Autodesk Inventor part; units mm, degrees
(part 2 of 2)
  arc A420 (-87.837, 33) -> (-86.5737, 31.4509) centre (-84.0686, 34.7833) ccw
  line L145 (-86.5737, 31.4509) -> (-85.9665, 30.9944)
  arc A421 (-84.6022, 29.6077) -> (-85.9665, 30.9944) centre (-89.9051, 25.7549) ccw
  arc A422 (-85.8476, 25.7748) -> (-84.6022, 29.6077) centre (-86.6173, 28.1437) ccw
  arc A423 (-87.7664, 25.4548) -> (-85.8476, 25.7748) centre (-87.8731, 32.0088) ccw
  line L146 (-87.7664, 25.4548) -> (-88.5259, 25.4425)
  arc A424 (-88.5259, 25.4425) -> (-90.4585, 24.9317) centre (-88.458, 21.274) ccw
  arc A425 (-90.4585, 24.9317) -> (-90.8052, 23.6378) centre (0, 0) ccw
  arc A426 (-90.8052, 23.6378) -> (-89.3869, 22.2292) centre (-87.2439, 25.8052) ccw
  line L147 (-89.3869, 22.2292) -> (-88.7353, 21.8387)
  arc A427 (-87.2336, 20.6022) -> (-88.7353, 21.8387) centre (-92.1048, 16.2162) ccw
  arc A428 (-88.0715, 16.6601) -> (-87.2336, 20.6022) centre (-89.0846, 18.9355) ccw
  arc A429 (-89.9463, 16.1413) -> (-88.0715, 16.6601) centre (-90.7376, 22.6482) ccw
  line L148 (-89.9463, 16.1413) -> (-90.7004, 16.0496)
  arc A430 (-90.7004, 16.0496) -> (-92.5691, 15.3396) centre (-90.1972, 11.9111) ccw
  arc A431 (-92.5691, 15.3396) -> (-92.7786, 14.0166) centre (0, 0) ccw
  arc A432 (-92.7786, 14.0166) -> (-91.2209, 12.7639) centre (-89.4633, 16.5444) ccw
  line L149 (-91.2209, 12.7639) -> (-90.532, 12.4437)
  arc A433 (-88.9092, 11.3709) -> (-90.532, 12.4437) centre (-93.2953, 6.4998) ccw
  arc A434 (-89.3305, 7.3628) -> (-88.9092, 11.3709) centre (-90.5759, 9.5199) ccw
  arc A435 (-91.1408, 6.6509) -> (-89.3305, 7.3628) centre (-92.6079, 13.0394) ccw
  line L150 (-91.1408, 6.6509) -> (-91.8812, 6.4809)
  arc A436 (-91.8812, 6.4809) -> (-93.6654, 5.5795) centre (-90.9481, 2.4177) ccw
  arc A437 (-93.6654, 5.5795) -> (-93.7355, 4.2418) centre (0, 0) ccw
  arc A438 (-93.7355, 4.2418) -> (-92.0553, 3.1588) centre (-90.7026, 7.1023) ccw
  line L151 (-92.0553, 3.1588) -> (-91.3368, 2.9123)
  arc A439 (-89.6108, 2.0151) -> (-91.3368, 2.9123) centre (-93.4636, -3.2878) ccw
  arc A440 (-89.6108, -2.0151) -> (-89.6108, 2.0151) centre (-91.0748, 0) ccw
  arc A441 (-91.3368, -2.9123) -> (-89.6108, -2.0151) centre (-93.4636, 3.2878) ccw
  line L152 (-91.3368, -2.9123) -> (-92.0553, -3.1588)
  arc A442 (-92.0553, -3.1588) -> (-93.7355, -4.2418) centre (-90.7026, -7.1023) ccw
  arc A443 (-93.7355, -4.2418) -> (-93.6654, -5.5795) centre (0, 0) ccw
  arc A444 (-93.6654, -5.5795) -> (-91.8812, -6.4809) centre (-90.9481, -2.4177) ccw
  line L153 (-91.8812, -6.4809) -> (-91.1408, -6.6509)
  arc A445 (-89.3305, -7.3628) -> (-91.1408, -6.6509) centre (-92.6079, -13.0394) ccw
  arc A446 (-88.9092, -11.3709) -> (-89.3305, -7.3628) centre (-90.5759, -9.5199) ccw
  arc A447 (-90.532, -12.4437) -> (-88.9092, -11.3709) centre (-93.2953, -6.4998) ccw
  line L154 (-90.532, -12.4437) -> (-91.2208, -12.7639)
  arc A448 (-91.2208, -12.7639) -> (-92.7786, -14.0166) centre (-89.4633, -16.5443) ccw
  arc A449 (-92.7786, -14.0166) -> (-92.5691, -15.3396) centre (0, 0) ccw
  arc A450 (-92.5691, -15.3396) -> (-90.7004, -16.0496) centre (-90.1972, -11.9111) ccw
  line L155 (-90.7004, -16.0496) -> (-89.9463, -16.1413)
  arc A451 (-88.0715, -16.6601) -> (-89.9463, -16.1413) centre (-90.7376, -22.6482) ccw
  arc A452 (-87.2336, -20.6022) -> (-88.0715, -16.6601) centre (-89.0846, -18.9355) ccw
  arc A453 (-88.7353, -21.8387) -> (-87.2336, -20.6022) centre (-92.1048, -16.2162) ccw
  line L156 (-88.7353, -21.8387) -> (-89.3869, -22.2292)
  arc A454 (-89.3869, -22.2292) -> (-90.8052, -23.6378) centre (-87.2439, -25.8052) ccw
  arc A455 (-90.8052, -23.6378) -> (-90.4585, -24.9317) centre (0, 0) ccw
  arc A456 (-90.4585, -24.9317) -> (-88.5259, -25.4425) centre (-88.458, -21.274) ccw
  line L157 (-88.5259, -25.4425) -> (-87.7664, -25.4548)
  arc A457 (-85.8476, -25.7748) -> (-87.7664, -25.4548) centre (-87.8732, -32.0088) ccw
  arc A458 (-84.6022, -29.6077) -> (-85.8476, -25.7748) centre (-86.6173, -28.1437) ccw
  arc A459 (-85.9665, -30.9944) -> (-84.6022, -29.6077) centre (-89.9052, -25.7549) ccw
  line L158 (-85.9665, -30.9944) -> (-86.5737, -31.4509)
  arc A460 (-86.5737, -31.4509) -> (-87.837, -33) centre (-84.0686, -34.7833) ccw
  arc A461 (-87.837, -33) -> (-87.3569, -34.2506) centre (0, 0) ccw
  arc A462 (-87.3569, -34.2506) -> (-85.3815, -34.5566) centre (-85.7497, -30.4038) ccw
  line L159 (-85.3815, -34.5566) -> (-84.6248, -34.4895)
  arc A463 (-82.6831, -34.6071) -> (-84.6248, -34.4895) centre (-84.0459, -41.0187) ccw
  arc A464 (-81.0439, -38.2889) -> (-82.6831, -34.6071) centre (-83.201, -37.0435) ccw
  arc A465 (-82.2557, -39.8105) -> (-81.0439, -38.2889) centre (-86.7205, -35.0115) ccw
  line L160 (-82.2557, -39.8105) -> (-82.8119, -40.328)
  arc A466 (-82.8119, -40.328) -> (-83.9063, -42.0007) centre (-79.9722, -43.3803) ccw
  arc A467 (-83.9063, -42.0007) -> (-83.2982, -43.1942) centre (0, 0) ccw
  arc A468 (-83.2982, -43.1942) -> (-81.3017, -43.2921) centre (-82.1019, -39.2006) ccw
  line L161 (-81.3017, -43.2921) -> (-80.5561, -43.1462)
  arc A469 (-78.6128, -43.0603) -> (-80.5561, -43.1462) centre (-79.2979, -49.5791) ccw
  arc A470 (-76.5977, -46.5505) -> (-78.6128, -43.0603) centre (-78.8731, -45.5374) ccw
  arc A471 (-77.6438, -48.1905) -> (-76.5977, -46.5505) centre (-82.5858, -43.8844) ccw
  line L162 (-77.6438, -48.1905) -> (-78.1428, -48.7633)
  arc A472 (-78.1428, -48.7633) -> (-79.0564, -50.5412) centre (-74.9996, -51.502) ccw
  arc A473 (-79.0564, -50.5412) -> (-78.3269, -51.6647) centre (0, 0) ccw
  arc A474 (-78.3269, -51.6647) -> (-76.331, -51.5532) centre (-77.5546, -47.5678) ccw
  line L163 (-76.331, -51.5532) -> (-75.6048, -51.3303)
  arc A475 (-73.6811, -51.0416) -> (-75.6048, -51.3303) centre (-73.6811, -57.5964) ccw
  arc A476 (-71.3122, -54.3021) -> (-73.6811, -51.0416) centre (-73.6811, -53.5324) ccw
  arc A477 (-72.1812, -56.0425) -> (-71.3122, -54.3021) centre (-77.5462, -52.2766) ccw
  line L164 (-72.1812, -56.0425) -> (-72.6176, -56.6643)
  arc A478 (-72.6176, -56.6643) -> (-73.3403, -58.528) centre (-69.2054, -59.0595) ccw
  arc A479 (-73.3403, -58.528) -> (-72.4974, -59.569) centre (0, 0) ccw
  arc A480 (-72.4974, -59.569) -> (-70.5241, -59.2496) centre (-72.1575, -55.4139) ccw
  line L165 (-70.5241, -59.2496) -> (-69.8252, -58.9519)
  arc A481 (-67.9421, -58.4638) -> (-69.8252, -58.9519) centre (-67.257, -64.9827) ccw
  arc A482 (-65.2454, -61.4588) -> (-67.9421, -58.4638) centre (-67.6818, -60.9409) ccw
  arc A483 (-65.9277, -63.2805) -> (-65.2454, -61.4588) centre (-71.657, -60.096) ccw
  line L166 (-65.9277, -63.2805) -> (-66.2968, -63.9445)
  arc A484 (-66.2968, -63.9445) -> (-66.8207, -65.8735) centre (-62.6528, -65.9699) ccw
  arc A485 (-66.8207, -65.8735) -> (-65.8735, -66.8207) centre (0, 0) ccw
  arc A486 (-65.8735, -66.8207) -> (-63.9445, -66.2968) centre (-65.9699, -62.6528) ccw
  line L167 (-63.9445, -66.2968) -> (-63.2805, -65.9277)
  arc A487 (-61.4588, -65.2454) -> (-63.2805, -65.9277) centre (-60.096, -71.657) ccw
  arc A488 (-58.4638, -67.9421) -> (-61.4588, -65.2454) centre (-60.941, -67.6818) ccw
  arc A489 (-58.952, -69.8252) -> (-58.4638, -67.9421) centre (-64.9827, -67.257) ccw
  line L168 (-58.952, -69.8252) -> (-59.2496, -70.5241)
  arc A490 (-59.2496, -70.5241) -> (-59.569, -72.4973) centre (-55.4139, -72.1575) ccw
  arc A491 (-59.569, -72.4973) -> (-58.528, -73.3403) centre (0, 0) ccw
  arc A492 (-58.528, -73.3403) -> (-56.6643, -72.6176) centre (-59.0595, -69.2054) ccw
  line L169 (-56.6643, -72.6176) -> (-56.0425, -72.1812)
  arc A493 (-54.3021, -71.3122) -> (-56.0425, -72.1812) centre (-52.2766, -77.5462) ccw
  arc A494 (-51.0416, -73.6811) -> (-54.3021, -71.3122) centre (-53.5324, -73.6811) ccw
  arc A495 (-51.3303, -75.6048) -> (-51.0416, -73.6811) centre (-57.5964, -73.6811) ccw
  line L170 (-51.3303, -75.6048) -> (-51.5532, -76.331)
  arc A496 (-51.5532, -76.331) -> (-51.6647, -78.3269) centre (-47.5678, -77.5545) ccw
  arc A497 (-51.6647, -78.3269) -> (-50.5412, -79.0564) centre (0, 0) ccw
  arc A498 (-50.5412, -79.0564) -> (-48.7633, -78.1428) centre (-51.502, -74.9996) ccw
  line L171 (-48.7633, -78.1428) -> (-48.1905, -77.6438)
  arc A499 (-46.5505, -76.5976) -> (-48.1905, -77.6438) centre (-43.8844, -82.5858) ccw
  arc A500 (-43.0603, -78.6127) -> (-46.5505, -76.5976) centre (-45.5374, -78.8731) ccw
  arc A501 (-43.1462, -80.5561) -> (-43.0603, -78.6127) centre (-49.5792, -79.2979) ccw
  line L172 (-43.1462, -80.5561) -> (-43.2921, -81.3016)
  arc A502 (-43.2921, -81.3016) -> (-43.1943, -83.2982) centre (-39.2006, -82.1019) ccw
  arc A503 (-43.1943, -83.2982) -> (-42.0007, -83.9063) centre (0, 0) ccw
  arc A504 (-42.0007, -83.9063) -> (-40.328, -82.8119) centre (-43.3803, -79.9722) ccw
  line L173 (-40.328, -82.8119) -> (-39.8105, -82.2557)
  arc A505 (-38.2889, -81.0439) -> (-39.8105, -82.2557) centre (-35.0115, -86.7205) ccw
  arc A506 (-34.6071, -82.6831) -> (-38.2889, -81.0439) centre (-37.0435, -83.201) ccw
  arc A507 (-34.4895, -84.6248) -> (-34.6071, -82.6831) centre (-41.0187, -84.0459) ccw
  line L174 (-34.4895, -84.6248) -> (-34.5566, -85.3815)
  arc A508 (-34.5566, -85.3815) -> (-34.2506, -87.3569) centre (-30.4038, -85.7497) ccw
  arc A509 (-34.2506, -87.3569) -> (-33, -87.837) centre (0, 0) ccw
  arc A510 (-33, -87.837) -> (-31.4509, -86.5737) centre (-34.7833, -84.0686) ccw
  line L175 (-31.4509, -86.5737) -> (-30.9944, -85.9665)
  arc A511 (-29.6077, -84.6022) -> (-30.9944, -85.9665) centre (-25.7549, -89.9051) ccw
  arc A512 (-25.7748, -85.8476) -> (-29.6077, -84.6022) centre (-28.1437, -86.6173) ccw
  arc A513 (-25.4548, -87.7664) -> (-25.7748, -85.8476) centre (-32.0088, -87.8731) ccw
  line L176 (-25.4548, -87.7664) -> (-25.4425, -88.5259)
  arc A514 (-25.4425, -88.5259) -> (-24.9317, -90.4585) centre (-21.274, -88.458) ccw
  arc A515 (-24.9317, -90.4585) -> (-23.6378, -90.8052) centre (0, 0) ccw
  arc A516 (-23.6378, -90.8052) -> (-22.2292, -89.3869) centre (-25.8052, -87.2439) ccw
  line L177 (-22.2292, -89.3869) -> (-21.8387, -88.7353)
  arc A517 (-20.6022, -87.2336) -> (-21.8387, -88.7353) centre (-16.2162, -92.1048) ccw
  arc A518 (-16.6601, -88.0715) -> (-20.6022, -87.2336) centre (-18.9355, -89.0846) ccw
  arc A519 (-16.1413, -89.9463) -> (-16.6601, -88.0715) centre (-22.6482, -90.7376) ccw
  line L178 (-16.1413, -89.9463) -> (-16.0496, -90.7004)
  arc A520 (-16.0496, -90.7004) -> (-15.3396, -92.5691) centre (-11.9111, -90.1972) ccw
  arc A521 (-15.3396, -92.5691) -> (-14.0166, -92.7786) centre (0, 0) ccw
  arc A522 (-14.0166, -92.7786) -> (-12.7639, -91.2208) centre (-16.5444, -89.4633) ccw
  line L179 (-12.7639, -91.2208) -> (-12.4437, -90.532)
  arc A523 (-11.3709, -88.9092) -> (-12.4437, -90.532) centre (-6.4998, -93.2952) ccw
  arc A524 (-7.3628, -89.3305) -> (-11.3709, -88.9092) centre (-9.5199, -90.5759) ccw
  arc A525 (-6.6509, -91.1408) -> (-7.3628, -89.3305) centre (-13.0394, -92.6079) ccw
  line L180 (-6.6509, -91.1408) -> (-6.4809, -91.8812)
  arc A526 (-6.4809, -91.8812) -> (-5.5795, -93.6654) centre (-2.4177, -90.9481) ccw
  arc A527 (-5.5795, -93.6654) -> (-4.2418, -93.7355) centre (0, 0) ccw
  arc A528 (-4.2418, -93.7355) -> (-3.1588, -92.0553) centre (-7.1023, -90.7026) ccw
  line L181 (-3.1588, -92.0553) -> (-2.9123, -91.3367)
  arc A529 (-2.0151, -89.6108) -> (-2.9123, -91.3367) centre (3.2878, -93.4636) ccw
  arc A530 (2.0151, -89.6108) -> (-2.0151, -89.6108) centre (0, -91.0748) ccw
  arc A531 (2.9123, -91.3368) -> (2.0151, -89.6108) centre (-3.2879, -93.4636) ccw
  line L182 (2.9123, -91.3368) -> (3.1588, -92.0553)
  arc A532 (3.1588, -92.0553) -> (4.2418, -93.7355) centre (7.1022, -90.7026) ccw
  arc A533 (4.2418, -93.7355) -> (5.5795, -93.6654) centre (0, 0) ccw
  arc A534 (5.5795, -93.6654) -> (6.4809, -91.8812) centre (2.4177, -90.9481) ccw
  line L183 (6.4809, -91.8812) -> (6.6509, -91.1408)
  arc A535 (7.3628, -89.3305) -> (6.6509, -91.1408) centre (13.0394, -92.6079) ccw
  arc A536 (11.3709, -88.9092) -> (7.3628, -89.3305) centre (9.5199, -90.5759) ccw
  arc A537 (12.4436, -90.532) -> (11.3709, -88.9092) centre (6.4998, -93.2952) ccw
  line L184 (12.4436, -90.532) -> (12.7639, -91.2208)
  arc A538 (12.7639, -91.2208) -> (14.0166, -92.7786) centre (16.5443, -89.4633) ccw
  arc A539 (14.0166, -92.7786) -> (15.3396, -92.5691) centre (0, 0) ccw
  arc A540 (15.3396, -92.5691) -> (16.0496, -90.7004) centre (11.9111, -90.1972) ccw
  line L185 (16.0496, -90.7004) -> (16.1413, -89.9463)
  arc A541 (16.6601, -88.0715) -> (16.1413, -89.9463) centre (22.6482, -90.7376) ccw
  arc A542 (20.6022, -87.2336) -> (16.6601, -88.0715) centre (18.9355, -89.0846) ccw
  arc A543 (21.8387, -88.7353) -> (20.6022, -87.2336) centre (16.2162, -92.1048) ccw
  line L186 (21.8387, -88.7353) -> (22.2291, -89.3869)
  arc A544 (22.2291, -89.3869) -> (23.6378, -90.8052) centre (25.8052, -87.2439) ccw
  arc A545 (23.6378, -90.8052) -> (24.9317, -90.4585) centre (0, 0) ccw
  arc A546 (24.9317, -90.4585) -> (25.4424, -88.5259) centre (21.274, -88.458) ccw
  line L187 (25.4424, -88.5259) -> (25.4548, -87.7664)
  arc A547 (25.7748, -85.8476) -> (25.4548, -87.7664) centre (32.0088, -87.8731) ccw
  arc A548 (29.6077, -84.6022) -> (25.7748, -85.8476) centre (28.1437, -86.6173) ccw
  arc A549 (30.9944, -85.9665) -> (29.6077, -84.6022) centre (25.7549, -89.9051) ccw
  line L188 (30.9944, -85.9665) -> (31.4508, -86.5737)
  arc A550 (31.4508, -86.5737) -> (33, -87.837) centre (34.7833, -84.0686) ccw
  arc A551 (33, -87.837) -> (34.2506, -87.3569) centre (0, 0) ccw
  arc A552 (34.2506, -87.3569) -> (34.5566, -85.3815) centre (30.4038, -85.7497) ccw
  line L189 (34.5566, -85.3815) -> (34.4895, -84.6248)
  arc A553 (34.6071, -82.6831) -> (34.4895, -84.6248) centre (41.0187, -84.0459) ccw
  arc A554 (38.2889, -81.0439) -> (34.6071, -82.6831) centre (37.0435, -83.201) ccw
  arc A555 (39.8105, -82.2557) -> (38.2889, -81.0439) centre (35.0115, -86.7205) ccw
  line L190 (39.8105, -82.2557) -> (40.328, -82.8119)
  arc A556 (40.328, -82.8119) -> (42.0007, -83.9063) centre (43.3803, -79.9722) ccw
  arc A557 (42.0007, -83.9063) -> (43.1942, -83.2982) centre (0, 0) ccw
  arc A558 (43.1942, -83.2982) -> (43.292, -81.3017) centre (39.2006, -82.1019) ccw
  line L191 (43.292, -81.3017) -> (43.1462, -80.5561)
  arc A559 (43.0602, -78.6127) -> (43.1462, -80.5561) centre (49.5791, -79.2979) ccw
  arc A560 (46.5505, -76.5976) -> (43.0602, -78.6127) centre (45.5374, -78.8731) ccw
  arc A561 (48.1905, -77.6438) -> (46.5505, -76.5976) centre (43.8844, -82.5858) ccw
  line L192 (48.1905, -77.6438) -> (48.7633, -78.1428)
  arc A562 (48.7633, -78.1428) -> (50.5412, -79.0564) centre (51.502, -74.9996) ccw
  arc A563 (50.5412, -79.0564) -> (51.6646, -78.3269) centre (0, 0) ccw
  arc A564 (51.6646, -78.3269) -> (51.5532, -76.331) centre (47.5678, -77.5546) ccw
  line L193 (51.5532, -76.331) -> (51.3303, -75.6048)
  arc A565 (51.0416, -73.6811) -> (51.3303, -75.6048) centre (57.5964, -73.6811) ccw
  arc A566 (54.3021, -71.3122) -> (51.0416, -73.6811) centre (53.5324, -73.6811) ccw
  arc A567 (56.0425, -72.1812) -> (54.3021, -71.3122) centre (52.2766, -77.5462) ccw
  line L194 (56.0425, -72.1812) -> (56.6643, -72.6176)
  arc A568 (56.6643, -72.6176) -> (58.528, -73.3403) centre (59.0595, -69.2054) ccw
  arc A569 (58.528, -73.3403) -> (59.569, -72.4973) centre (0, 0) ccw
  arc A570 (59.569, -72.4973) -> (59.2496, -70.5241) centre (55.4139, -72.1575) ccw
  line L195 (59.2496, -70.5241) -> (58.9519, -69.8252)
  arc A571 (58.4638, -67.9421) -> (58.9519, -69.8252) centre (64.9827, -67.257) ccw
  arc A572 (61.4588, -65.2454) -> (58.4638, -67.9421) centre (60.9409, -67.6818) ccw
  arc A573 (63.2805, -65.9277) -> (61.4588, -65.2454) centre (60.096, -71.657) ccw
  line L196 (63.2805, -65.9277) -> (63.9445, -66.2968)
  arc A574 (63.9445, -66.2968) -> (65.8735, -66.8207) centre (65.9699, -62.6528) ccw
  arc A575 (65.8735, -66.8207) -> (66.8207, -65.8735) centre (0, 0) ccw
  arc A576 (66.8207, -65.8735) -> (66.2968, -63.9445) centre (62.6528, -65.9699) ccw
  line L197 (66.2968, -63.9445) -> (65.9277, -63.2805)
  arc A577 (65.2454, -61.4588) -> (65.9277, -63.2805) centre (71.657, -60.096) ccw
  arc A578 (67.9421, -58.4638) -> (65.2454, -61.4588) centre (67.6818, -60.941) ccw
  arc A579 (69.8252, -58.9519) -> (67.9421, -58.4638) centre (67.257, -64.9827) ccw
  line L198 (69.8252, -58.9519) -> (70.5241, -59.2496)
  arc A580 (70.5241, -59.2496) -> (72.4973, -59.569) centre (72.1575, -55.4139) ccw
  arc A581 (72.4973, -59.569) -> (73.3403, -58.528) centre (0, 0) ccw
  arc A582 (73.3403, -58.528) -> (72.6176, -56.6643) centre (69.2053, -59.0595) ccw
  line L199 (72.6176, -56.6643) -> (72.1812, -56.0425)
  arc A583 (71.3122, -54.3021) -> (72.1812, -56.0425) centre (77.5462, -52.2766) ccw
  arc A584 (73.6811, -51.0416) -> (71.3122, -54.3021) centre (73.6811, -53.5324) ccw
  arc A585 (75.6048, -51.3303) -> (73.6811, -51.0416) centre (73.6811, -57.5964) ccw
  line L200 (75.6048, -51.3303) -> (76.331, -51.5532)
  arc A586 (76.331, -51.5532) -> (78.3268, -51.6647) centre (77.5545, -47.5678) ccw
  arc A587 (78.3268, -51.6647) -> (79.0564, -50.5412) centre (0, 0) ccw
  arc A588 (79.0564, -50.5412) -> (78.1428, -48.7633) centre (74.9996, -51.502) ccw
  line L201 (78.1428, -48.7633) -> (77.6438, -48.1905)
  arc A589 (76.5976, -46.5505) -> (77.6438, -48.1905) centre (82.5857, -43.8844) ccw
  arc A590 (78.6127, -43.0603) -> (76.5976, -46.5505) centre (78.8731, -45.5374) ccw
  arc A591 (80.5561, -43.1462) -> (78.6127, -43.0603) centre (79.2979, -49.5791) ccw
  line L202 (80.5561, -43.1462) -> (81.3016, -43.2921)
  arc A592 (81.3016, -43.2921) -> (83.2982, -43.1943) centre (82.1019, -39.2006) ccw
  arc A593 (83.2982, -43.1943) -> (83.9063, -42.0007) centre (0, 0) ccw
  arc A594 (83.9063, -42.0007) -> (82.8119, -40.328) centre (79.9722, -43.3803) ccw
  line L203 (82.8119, -40.328) -> (82.2557, -39.8105)
  arc A595 (81.0439, -38.2889) -> (82.2557, -39.8105) centre (86.7205, -35.0115) ccw
  arc A596 (82.6831, -34.6071) -> (81.0439, -38.2889) centre (83.201, -37.0435) ccw
  arc A597 (84.6248, -34.4895) -> (82.6831, -34.6071) centre (84.0459, -41.0187) ccw
  line L204 (84.6248, -34.4895) -> (85.3815, -34.5566)
  arc A598 (85.3815, -34.5566) -> (87.3569, -34.2506) centre (85.7497, -30.4038) ccw
  arc A599 (87.3569, -34.2506) -> (87.837, -33) centre (0, 0) ccw
  arc A600 (87.837, -33) -> (86.5737, -31.4509) centre (84.0686, -34.7833) ccw
  line L205 (86.5737, -31.4509) -> (85.9664, -30.9944)
  arc A601 (84.6022, -29.6077) -> (85.9664, -30.9944) centre (89.9051, -25.7549) ccw
  arc A602 (85.8476, -25.7748) -> (84.6022, -29.6077) centre (86.6173, -28.1437) ccw
  arc A603 (87.7664, -25.4548) -> (85.8476, -25.7748) centre (87.8731, -32.0088) ccw
  line L206 (87.7664, -25.4548) -> (88.5259, -25.4425)
  arc A604 (88.5259, -25.4425) -> (90.4585, -24.9317) centre (88.458, -21.274) ccw
  arc A605 (90.4585, -24.9317) -> (90.8052, -23.6378) centre (0, 0) ccw
  arc A606 (90.8052, -23.6378) -> (89.3869, -22.2292) centre (87.2439, -25.8052) ccw
  line L207 (89.3869, -22.2292) -> (88.7353, -21.8387)
  arc A607 (87.2336, -20.6022) -> (88.7353, -21.8387) centre (92.1048, -16.2162) ccw
  arc A608 (88.0715, -16.6601) -> (87.2336, -20.6022) centre (89.0846, -18.9355) ccw
  arc A609 (89.9463, -16.1413) -> (88.0715, -16.6601) centre (90.7376, -22.6482) ccw
  line L208 (89.9463, -16.1413) -> (90.7004, -16.0496)
  arc A610 (90.7004, -16.0496) -> (92.569, -15.3396) centre (90.1972, -11.9111) ccw
  arc A611 (92.569, -15.3396) -> (92.7786, -14.0166) centre (0, 0) ccw
  arc A612 (92.7786, -14.0166) -> (91.2208, -12.7639) centre (89.4633, -16.5444) ccw
  line L209 (91.2208, -12.7639) -> (90.532, -12.4437)
  arc A613 (88.9092, -11.3709) -> (90.532, -12.4437) centre (93.2952, -6.4998) ccw
  arc A614 (89.3305, -7.3628) -> (88.9092, -11.3709) centre (90.5759, -9.5199) ccw
  arc A615 (91.1408, -6.6509) -> (89.3305, -7.3628) centre (92.6079, -13.0394) ccw
  line L210 (91.1408, -6.6509) -> (91.8812, -6.4809)
  arc A616 (91.8812, -6.4809) -> (93.6654, -5.5795) centre (90.9481, -2.4177) ccw
  arc A617 (93.6654, -5.5795) -> (93.7355, -4.2418) centre (0, 0) ccw
  arc A618 (93.7355, -4.2418) -> (92.0553, -3.1588) centre (90.7026, -7.1023) ccw
  line L211 (92.0553, -3.1588) -> (91.3367, -2.9123)
  arc A619 (89.6108, -2.0151) -> (91.3367, -2.9123) centre (93.4636, 3.2878) ccw
  arc A620 (89.6108, 2.0151) -> (89.6108, -2.0151) centre (91.0748, 0) ccw
  arc A621 (91.3368, 2.9123) -> (89.6108, 2.0151) centre (93.4636, -3.2878) ccw
  line L212 (91.3368, 2.9123) -> (92.0553, 3.1588)
  arc A622 (92.0553, 3.1588) -> (93.7355, 4.2418) centre (90.7026, 7.1022) ccw
  arc A623 (93.7355, 4.2418) -> (93.6654, 5.5795) centre (0, 0) ccw
  arc A624 (93.6654, 5.5795) -> (91.8812, 6.4809) centre (90.9481, 2.4177) ccw
  line L213 (91.8812, 6.4809) -> (91.1408, 6.6509)
  arc A625 (89.3305, 7.3628) -> (91.1408, 6.6509) centre (92.6079, 13.0394) ccw
  arc A626 (88.9092, 11.3709) -> (89.3305, 7.3628) centre (90.5759, 9.5199) ccw
  arc A627 (90.532, 12.4437) -> (88.9092, 11.3709) centre (93.2952, 6.4998) ccw
  line L214 (90.532, 12.4437) -> (91.2208, 12.7639)
  arc A628 (91.2208, 12.7639) -> (92.7786, 14.0166) centre (89.4633, 16.5443) ccw
  arc A629 (92.7786, 14.0166) -> (92.569, 15.3396) centre (0, 0) ccw
  arc A630 (92.569, 15.3396) -> (90.7004, 16.0496) centre (90.1972, 11.9111) ccw
  line L215 (90.7004, 16.0496) -> (89.9463, 16.1413)
  arc A631 (88.0715, 16.6601) -> (89.9463, 16.1413) centre (90.7376, 22.6482) ccw
  arc A632 (87.2336, 20.6022) -> (88.0715, 16.6601) centre (89.0846, 18.9355) ccw
  arc A633 (88.7353, 21.8387) -> (87.2336, 20.6022) centre (92.1048, 16.2162) ccw
  line L216 (88.7353, 21.8387) -> (89.3869, 22.2291)
  arc A634 (89.3869, 22.2291) -> (90.8052, 23.6378) centre (87.2439, 25.8052) ccw
  arc A635 (90.8052, 23.6378) -> (90.4585, 24.9317) centre (0, 0) ccw
  arc A636 (90.4585, 24.9317) -> (88.5259, 25.4425) centre (88.458, 21.274) ccw
  line L217 (88.5259, 25.4425) -> (87.7664, 25.4548)
  arc A637 (85.8476, 25.7748) -> (87.7664, 25.4548) centre (87.8731, 32.0088) ccw
  arc A638 (84.6022, 29.6077) -> (85.8476, 25.7748) centre (86.6173, 28.1437) ccw
  arc A639 (85.9665, 30.9944) -> (84.6022, 29.6077) centre (89.9051, 25.7549) ccw
  line L218 (85.9665, 30.9944) -> (86.5737, 31.4509)
  arc A640 (86.5737, 31.4509) -> (87.837, 33) centre (84.0686, 34.7833) ccw
  arc A641 (87.837, 33) -> (87.3569, 34.2506) centre (0, 0) ccw
  arc A642 (87.3569, 34.2506) -> (85.3815, 34.5566) centre (85.7497, 30.4038) ccw
  line L219 (85.3815, 34.5566) -> (84.6248, 34.4895)
  arc A643 (82.6831, 34.6071) -> (84.6248, 34.4895) centre (84.0459, 41.0187) ccw
  arc A644 (81.0439, 38.2889) -> (82.6831, 34.6071) centre (83.201, 37.0435) ccw
  arc A645 (82.2557, 39.8105) -> (81.0439, 38.2889) centre (86.7205, 35.0115) ccw
  line L220 (82.2557, 39.8105) -> (82.8119, 40.328)
  arc A646 (82.8119, 40.328) -> (83.9063, 42.0007) centre (79.9722, 43.3803) ccw
  arc A647 (83.9063, 42.0007) -> (83.2982, 43.1942) centre (0, 0) ccw
  arc A648 (83.2982, 43.1942) -> (81.3016, 43.2921) centre (82.1019, 39.2006) ccw
  line L221 (81.3016, 43.2921) -> (80.5561, 43.1462)
  arc A649 (78.6127, 43.0603) -> (80.5561, 43.1462) centre (79.2979, 49.5791) ccw
  arc A650 (76.5976, 46.5505) -> (78.6127, 43.0603) centre (78.8731, 45.5374) ccw
  arc A651 (77.6438, 48.1905) -> (76.5976, 46.5505) centre (82.5858, 43.8844) ccw
  line L222 (77.6438, 48.1905) -> (78.1428, 48.7633)
  arc A652 (78.1428, 48.7633) -> (79.0564, 50.5412) centre (74.9996, 51.502) ccw
  arc A653 (79.0564, 50.5412) -> (78.3269, 51.6647) centre (0, 0) ccw
  arc A654 (78.3269, 51.6647) -> (76.331, 51.5532) centre (77.5545, 47.5678) ccw
  line L223 (76.331, 51.5532) -> (75.6048, 51.3303)
  arc A655 (73.6811, 51.0416) -> (75.6048, 51.3303) centre (73.6811, 57.5964) ccw
  arc A656 (71.3122, 54.3021) -> (73.6811, 51.0416) centre (73.6811, 53.5324) ccw
  arc A657 (72.1812, 56.0425) -> (71.3122, 54.3021) centre (77.5462, 52.2766) ccw
  line L224 (72.1812, 56.0425) -> (72.6176, 56.6643)
  arc A658 (72.6176, 56.6643) -> (73.3403, 58.528) centre (69.2053, 59.0595) ccw
  arc A659 (73.3403, 58.528) -> (72.4973, 59.569) centre (0, 0) ccw
  arc A660 (72.4973, 59.569) -> (70.5241, 59.2496) centre (72.1575, 55.4139) ccw
  line L225 (70.5241, 59.2496) -> (69.8251, 58.9519)
  arc A661 (67.9421, 58.4638) -> (69.8251, 58.9519) centre (67.257, 64.9827) ccw
  arc A662 (65.2454, 61.4588) -> (67.9421, 58.4638) centre (67.6818, 60.9409) ccw
  arc A663 (65.9277, 63.2805) -> (65.2454, 61.4588) centre (71.657, 60.096) ccw
  line L226 (65.9277, 63.2805) -> (66.2968, 63.9445)
  arc A664 (66.2968, 63.9445) -> (66.8207, 65.8735) centre (62.6528, 65.9699) ccw
  arc A665 (66.8207, 65.8735) -> (65.8735, 66.8207) centre (0, 0) ccw
  arc A666 (65.8735, 66.8207) -> (63.9445, 66.2968) centre (65.9699, 62.6528) ccw
  line L227 (63.9445, 66.2968) -> (63.2805, 65.9277)
  arc A667 (61.4588, 65.2454) -> (63.2805, 65.9277) centre (60.096, 71.657) ccw
  arc A668 (58.4638, 67.9421) -> (61.4588, 65.2454) centre (60.9409, 67.6818) ccw
  arc A669 (58.9519, 69.8252) -> (58.4638, 67.9421) centre (64.9827, 67.257) ccw
  line L228 (58.9519, 69.8252) -> (59.2496, 70.5241)
  arc A670 (59.2496, 70.5241) -> (59.569, 72.4973) centre (55.4139, 72.1575) ccw
  arc A671 (59.569, 72.4973) -> (58.528, 73.3403) centre (0, 0) ccw
  arc A672 (58.528, 73.3403) -> (56.6643, 72.6176) centre (59.0595, 69.2053) ccw
  line L229 (56.6643, 72.6176) -> (56.0425, 72.1812)
  arc A673 (54.3021, 71.3122) -> (56.0425, 72.1812) centre (52.2766, 77.5462) ccw
  arc A674 (51.0416, 73.6811) -> (54.3021, 71.3122) centre (53.5324, 73.6811) ccw
  arc A675 (51.3303, 75.6048) -> (51.0416, 73.6811) centre (57.5964, 73.6811) ccw
  line L230 (51.3303, 75.6048) -> (51.5532, 76.331)
  arc A676 (51.5532, 76.331) -> (51.6647, 78.3269) centre (47.5678, 77.5545) ccw
  arc A677 (51.6647, 78.3269) -> (50.5412, 79.0564) centre (0, 0) ccw
  arc A678 (50.5412, 79.0564) -> (48.7633, 78.1428) centre (51.502, 74.9996) ccw
  line L231 (48.7633, 78.1428) -> (48.1905, 77.6438)
  arc A679 (46.5505, 76.5976) -> (48.1905, 77.6438) centre (43.8844, 82.5858) ccw
  arc A680 (43.0603, 78.6127) -> (46.5505, 76.5976) centre (45.5374, 78.8731) ccw
  arc A681 (43.1462, 80.5561) -> (43.0603, 78.6127) centre (49.5791, 79.2979) ccw
  line L232 (43.1462, 80.5561) -> (43.292, 81.3016)
  arc A682 (43.292, 81.3016) -> (43.1942, 83.2982) centre (39.2006, 82.1019) ccw
  arc A683 (43.1942, 83.2982) -> (42.0007, 83.9063) centre (0, 0) ccw
  arc A684 (42.0007, 83.9063) -> (40.328, 82.8119) centre (43.3803, 79.9722) ccw
  line L233 (40.328, 82.8119) -> (39.8105, 82.2557)
  arc A685 (38.2889, 81.0439) -> (39.8105, 82.2557) centre (35.0115, 86.7205) ccw
  arc A686 (34.6071, 82.6831) -> (38.2889, 81.0439) centre (37.0435, 83.201) ccw
  arc A687 (34.4895, 84.6248) -> (34.6071, 82.6831) centre (41.0187, 84.0459) ccw
  line L234 (34.4895, 84.6248) -> (34.5566, 85.3815)
  arc A688 (34.5566, 85.3815) -> (34.2506, 87.3569) centre (30.4038, 85.7497) ccw
  arc A689 (34.2506, 87.3569) -> (33, 87.837) centre (0, 0) ccw
  arc A690 (33, 87.837) -> (31.4509, 86.5737) centre (34.7833, 84.0686) ccw
  line L235 (31.4509, 86.5737) -> (30.9944, 85.9665)
  arc A691 (29.6077, 84.6022) -> (30.9944, 85.9665) centre (25.7549, 89.9051) ccw
  arc A692 (25.7748, 85.8476) -> (29.6077, 84.6022) centre (28.1437, 86.6173) ccw
  arc A693 (25.4548, 87.7664) -> (25.7748, 85.8476) centre (32.0088, 87.8731) ccw
  line L236 (25.4548, 87.7664) -> (25.4425, 88.5259)
  arc A694 (25.4425, 88.5259) -> (24.9317, 90.4585) centre (21.274, 88.458) ccw
  arc A695 (24.9317, 90.4585) -> (23.6378, 90.8052) centre (0, 0) ccw
  arc A696 (23.6378, 90.8052) -> (22.2292, 89.3869) centre (25.8052, 87.2439) ccw
  line L237 (22.2292, 89.3869) -> (21.8386, 88.7353)
  arc A697 (20.6022, 87.2336) -> (21.8386, 88.7353) centre (16.2162, 92.1048) ccw
  arc A698 (16.6601, 88.0715) -> (20.6022, 87.2336) centre (18.9355, 89.0846) ccw
  arc A699 (16.1413, 89.9463) -> (16.6601, 88.0715) centre (22.6482, 90.7376) ccw
  line L238 (16.1413, 89.9463) -> (16.0496, 90.7004)
  arc A700 (16.0496, 90.7004) -> (15.3396, 92.5691) centre (11.9111, 90.1972) ccw
  arc A701 (15.3396, 92.5691) -> (14.0166, 92.7786) centre (0, 0) ccw
  arc A702 (14.0166, 92.7786) -> (12.7639, 91.2208) centre (16.5443, 89.4633) ccw
  line L239 (12.7639, 91.2208) -> (12.4436, 90.532)
  arc A703 (11.3709, 88.9092) -> (12.4436, 90.532) centre (6.4998, 93.2952) ccw
  arc A704 (7.3628, 89.3305) -> (11.3709, 88.9092) centre (9.5199, 90.5759) ccw
  arc A705 (6.6509, 91.1408) -> (7.3628, 89.3305) centre (13.0394, 92.6079) ccw
  line L240 (6.6509, 91.1408) -> (6.4809, 91.8812)
  arc A706 (6.4809, 91.8812) -> (5.5795, 93.6654) centre (2.4177, 90.9481) ccw
  arc A707 (5.5795, 93.6654) -> (4.2418, 93.7355) centre (0, 0) ccw
  arc A708 (4.2418, 93.7355) -> (3.1588, 92.0553) centre (7.1022, 90.7026) ccw
  line L241 (3.1588, 92.0553) -> (2.9123, 91.3367)
  arc A709 (2.0151, 89.6108) -> (2.9123, 91.3367) centre (-3.2878, 93.4636) ccw
  arc A710 (-2.0151, 89.6108) -> (2.0151, 89.6108) centre (0, 91.0748) ccw
  arc A711 (-2.9123, 91.3368) -> (-2.0151, 89.6108) centre (3.2878, 93.4636) ccw
  line L242 (-2.9123, 91.3368) -> (-3.1588, 92.0553)
  arc A712 (-3.1588, 92.0553) -> (-4.2418, 93.7355) centre (-7.1023, 90.7026) ccw
  arc A713 (-4.2418, 93.7355) -> (-5.5795, 93.6654) centre (0, 0) ccw
  arc A714 (-5.5795, 93.6654) -> (-6.4809, 91.8812) centre (-2.4177, 90.9481) ccw
  line L243 (-6.4809, 91.8812) -> (-6.6509, 91.1408)
  arc A715 (-7.3628, 89.3305) -> (-6.6509, 91.1408) centre (-13.0394, 92.6079) ccw
  arc A716 (-11.3709, 88.9092) -> (-7.3628, 89.3305) centre (-9.5199, 90.5759) ccw
  arc A717 (-12.4437, 90.532) -> (-11.3709, 88.9092) centre (-6.4998, 93.2952) ccw
  line L244 (-12.4437, 90.532) -> (-12.7639, 91.2208)
  arc A718 (-12.7639, 91.2208) -> (-14.0166, 92.7786) centre (-16.5444, 89.4633) ccw
  arc A719 (-14.0166, 92.7786) -> (-15.3396, 92.5691) centre (0, 0) ccw
  arc A720 (-15.3396, 92.5691) -> (-16.0496, 90.7004) centre (-11.9111, 90.1972) ccw
  line L245 (-16.0496, 90.7004) -> (-16.1413, 89.9463)
  arc A721 (-16.6601, 88.0715) -> (-16.1413, 89.9463) centre (-22.6482, 90.7376) ccw
  arc A722 (-20.6022, 87.2336) -> (-16.6601, 88.0715) centre (-18.9355, 89.0846) ccw
  arc A723 (-21.8387, 88.7353) -> (-20.6022, 87.2336) centre (-16.2162, 92.1048) ccw
  line L246 (-21.8387, 88.7353) -> (-22.2292, 89.3869)
  arc A724 (-22.2292, 89.3869) -> (-23.6378, 90.8052) centre (-25.8052, 87.2439) ccw
  arc A725 (-23.6378, 90.8052) -> (-24.9317, 90.4585) centre (0, 0) ccw
  arc A726 (-24.9317, 90.4585) -> (-25.4425, 88.5259) centre (-21.274, 88.458) ccw
  line L247 (-25.4425, 88.5259) -> (-25.4548, 87.7664)
  arc A727 (-25.7748, 85.8476) -> (-25.4548, 87.7664) centre (-32.0088, 87.8731) ccw
  arc A728 (-29.6077, 84.6022) -> (-25.7748, 85.8476) centre (-28.1437, 86.6173) ccw
  arc A729 (-30.9944, 85.9665) -> (-29.6077, 84.6022) centre (-25.7549, 89.9051) ccw
  line L248 (-30.9944, 85.9665) -> (-31.4509, 86.5737)
  arc A730 (-31.4509, 86.5737) -> (-33, 87.837) centre (-34.7833, 84.0686) ccw
  arc A731 (-33, 87.837) -> (-34.2506, 87.3569) centre (0, 0) ccw
  arc A732 (-34.2506, 87.3569) -> (-34.5566, 85.3815) centre (-30.4038, 85.7497) ccw
  line L249 (-34.5566, 85.3815) -> (-34.4895, 84.6248)
  arc A733 (-34.6071, 82.6831) -> (-34.4895, 84.6248) centre (-41.0187, 84.0459) ccw
  arc A734 (-38.2889, 81.0439) -> (-34.6071, 82.6831) centre (-37.0435, 83.201) ccw
  arc A735 (-39.8105, 82.2557) -> (-38.2889, 81.0439) centre (-35.0115, 86.7205) ccw
  line L250 (-39.8105, 82.2557) -> (-40.328, 82.8119)
  arc A736 (-40.328, 82.8119) -> (-42.0007, 83.9063) centre (-43.3803, 79.9722) ccw
  arc A737 (-42.0007, 83.9063) -> (-43.1943, 83.2982) centre (0, 0) ccw
  arc A738 (-43.1943, 83.2982) -> (-43.2921, 81.3016) centre (-39.2006, 82.1019) ccw
  line L251 (-43.2921, 81.3016) -> (-43.1462, 80.5561)
  arc A739 (-43.0603, 78.6127) -> (-43.1462, 80.5561) centre (-49.5792, 79.2979) ccw
  arc A740 (-46.5505, 76.5976) -> (-43.0603, 78.6127) centre (-45.5374, 78.8731) ccw
  arc A741 (-48.1905, 77.6438) -> (-46.5505, 76.5976) centre (-43.8844, 82.5858) ccw
  line L252 (-48.1905, 77.6438) -> (-48.7633, 78.1428)
  arc A742 (-48.7633, 78.1428) -> (-50.5412, 79.0564) centre (-51.502, 74.9996) ccw
  arc A743 (-50.5412, 79.0564) -> (-51.6647, 78.3269) centre (0, 0) ccw
  arc A744 (-51.6647, 78.3269) -> (-51.5532, 76.331) centre (-47.5678, 77.5545) ccw
  line L253 (-51.5532, 76.331) -> (-51.3303, 75.6048)
  arc A745 (-51.0416, 73.6811) -> (-51.3303, 75.6048) centre (-57.5964, 73.6811) ccw
  arc A746 (-54.3021, 71.3122) -> (-51.0416, 73.6811) centre (-53.5324, 73.6811) ccw
  arc A747 (-56.0425, 72.1812) -> (-54.3021, 71.3122) centre (-52.2766, 77.5462) ccw
  line L254 (-56.0425, 72.1812) -> (-56.6643, 72.6176)
  arc A748 (-56.6643, 72.6176) -> (-58.528, 73.3403) centre (-59.0595, 69.2053) ccw
  arc A749 (-58.528, 73.3403) -> (-59.569, 72.4973) centre (0, 0) ccw
  arc A750 (-59.569, 72.4973) -> (-59.2496, 70.5241) centre (-55.4139, 72.1575) ccw
  line L255 (-59.2496, 70.5241) -> (-58.9519, 69.8252)
  arc A751 (-58.4638, 67.9421) -> (-58.9519, 69.8252) centre (-64.9827, 67.257) ccw
  arc A752 (-61.4588, 65.2454) -> (-58.4638, 67.9421) centre (-60.941, 67.6818) ccw
  arc A753 (-63.2805, 65.9277) -> (-61.4588, 65.2454) centre (-60.096, 71.657) ccw
  line L256 (-63.2805, 65.9277) -> (-63.9445, 66.2968)
  arc A754 (-63.9445, 66.2968) -> (-65.8735, 66.8207) centre (-65.9699, 62.6528) ccw
  arc A755 (-65.8735, 66.8207) -> (-66.8207, 65.8735) centre (0, 0) ccw
  arc A756 (-66.8207, 65.8735) -> (-66.2968, 63.9445) centre (-62.6528, 65.9699) ccw
  line L257 (-66.2968, 63.9445) -> (-65.9277, 63.2805)
  arc A757 (-65.2454, 61.4588) -> (-65.9277, 63.2805) centre (-71.657, 60.096) ccw
  arc A758 (-67.9421, 58.4638) -> (-65.2454, 61.4588) centre (-67.6818, 60.9409) ccw
  arc A759 (-69.8252, 58.9519) -> (-67.9421, 58.4638) centre (-67.257, 64.9827) ccw
  line L258 (-69.8252, 58.9519) -> (-70.5241, 59.2496)
  arc A760 (-70.5241, 59.2496) -> (-72.4974, 59.569) centre (-72.1575, 55.4139) ccw
  arc A761 (-72.4974, 59.569) -> (-73.3403, 58.528) centre (0, 0) ccw
  arc A762 (-73.3403, 58.528) -> (-72.6176, 56.6643) centre (-69.2054, 59.0595) ccw
  line L259 (-72.6176, 56.6643) -> (-72.1812, 56.0425)
  dimension "d6" = 0.1
  constraints: 1512 point on circle, 763 centre point, 516 end point, 2 collinear, 2 midpoint, 2 parallel, 1 horizontal, 1 perpendicular, 1945 other
  measures "d6" radial gap between concentric circles of A49 A761
extrude "Extrusion2" add sketch "Sketch2" along normal mid plane 6.35
sketch "Sketch3" plane through (0, 0, 0) normal (0, 0, -1) x (-1, 0, 0)
  circle A0 centre (0, 0) radius 63.5
  dimension "d7" = 127
  constraints: 1 centre point, 1 coincident
  measures "d7" diameter of A0
extrude "Extrusion3" cut sketch "Sketch3" against normal blind 6.35
sketch "Sketch4" plane through (0, 0, -5.3215) normal (0, 0, -1) x (-1, 0, 0)
  circle A0 centre (-88.9, 88.9) radius 3.175
  line L0 (-101.6, 101.6) -> (-101.6, -101.6) projected
  line L1 (101.6, 101.6) -> (-101.6, 101.6) projected
  circle A1 centre (-76.2, 88.9) radius 3.175
  circle A2 centre (-88.9, 76.2) radius 3.175
  circle A3 centre (-76.2, 76.2) radius 3.175
  circle A4 centre (-63.5, 88.9) radius 3.175
  circle A5 centre (-63.5, 76.2) radius 3.175
  circle A6 centre (-50.8, 88.9) radius 3.175
  circle A7 centre (-50.8, 76.2) radius 3.175
  circle A8 centre (-88.9, 63.5) radius 3.175
  circle A9 centre (-76.2, 63.5) radius 3.175
  circle A10 centre (-63.5, 63.5) radius 3.175
  circle A11 centre (-50.8, 63.5) radius 3.175
  circle A12 centre (-88.9, 50.8) radius 3.175
  circle A13 centre (-76.2, 50.8) radius 3.175
  circle A14 centre (-63.5, 50.8) radius 3.175
  circle A15 centre (-50.8, 50.8) radius 3.175
  circle A16 centre (-63.5, -63.5) radius 3.175
  circle A17 centre (-76.2, -63.5) radius 3.175
  circle A18 centre (-88.9, -63.5) radius 3.175
  circle A19 centre (-88.9, -50.8) radius 3.175
  circle A20 centre (-76.2, -50.8) radius 3.175
  circle A21 centre (-50.8, -50.8) radius 3.175
  circle A22 centre (-63.5, -50.8) radius 3.175
  circle A23 centre (-50.8, -76.2) radius 3.175
  circle A24 centre (-63.5, -76.2) radius 3.175
  circle A25 centre (-76.2, -76.2) radius 3.175
  circle A26 centre (-50.8, -88.9) radius 3.175
  circle A27 centre (-63.5, -88.9) radius 3.175
  circle A28 centre (-88.9, -76.2) radius 3.175
  circle A29 centre (-76.2, -88.9) radius 3.175
  circle A30 centre (-88.9, -88.9) radius 3.175
  circle A31 centre (-50.8, -63.5) radius 3.175
  circle A32 centre (63.5, -63.5) radius 3.175
  circle A33 centre (63.5, -76.2) radius 3.175
  circle A34 centre (63.5, -88.9) radius 3.175
  circle A35 centre (50.8, -88.9) radius 3.175
  circle A36 centre (50.8, -76.2) radius 3.175
  circle A37 centre (50.8, -50.8) radius 3.175
  circle A38 centre (50.8, -63.5) radius 3.175
  circle A39 centre (76.2, -50.8) radius 3.175
  circle A40 centre (76.2, -63.5) radius 3.175
  circle A41 centre (76.2, -76.2) radius 3.175
  circle A42 centre (88.9, -50.8) radius 3.175
  circle A43 centre (88.9, -63.5) radius 3.175
  circle A44 centre (76.2, -88.9) radius 3.175
  circle A45 centre (88.9, -76.2) radius 3.175
  circle A46 centre (88.9, -88.9) radius 3.175
  circle A47 centre (63.5, -50.8) radius 3.175
  circle A48 centre (63.5, 63.5) radius 3.175
  circle A49 centre (76.2, 63.5) radius 3.175
  circle A50 centre (88.9, 63.5) radius 3.175
  circle A51 centre (88.9, 50.8) radius 3.175
  circle A52 centre (76.2, 50.8) radius 3.175
  circle A53 centre (50.8, 50.8) radius 3.175
  circle A54 centre (63.5, 50.8) radius 3.175
  circle A55 centre (50.8, 76.2) radius 3.175
  circle A56 centre (63.5, 76.2) radius 3.175
  circle A57 centre (76.2, 76.2) radius 3.175
  circle A58 centre (50.8, 88.9) radius 3.175
  circle A59 centre (63.5, 88.9) radius 3.175
  circle A60 centre (88.9, 76.2) radius 3.175
  circle A61 centre (76.2, 88.9) radius 3.175
  circle A62 centre (88.9, 88.9) radius 3.175
  circle A63 centre (50.8, 63.5) radius 3.175
  point P0 (0, 0)
  dimension "d10" = 12.7
  dimension "d11" = 12.7
  dimension "d12" = 6.35
  dimension "d15" = 12.7
  dimension "d18" = 12.7
  dimension "d25" = 360
  constraints: 64 centre point, 1 horizontal, 1 vertical, 159 other
  measures "d10" distance from line of A0.centre L0
  measures "d11" distance from line of A0.centre L1
  measures "d12" diameter of A0
  measures "d15" distance of A0.centre A1.centre
  measures "d18" distance of A0.centre A2.centre
extrude "Extrusion4" cut sketch "Sketch4" against normal through all contours A0 | A1 | A2 | A3 | A4 | A5 | A6 | A8 | A9 | A12 | A17 | A18 | A19 | A24 | A25 | A26 | A27 | A28 | A29 | A30 | A33 | A34 | A35 | A40 | A41 | A42 | A43 | A44 | A45 | A46 | A49 | A50 | A51 | A56 | A57 | A58 | A59 | A60 | A61 | A62
body "Solid1"
